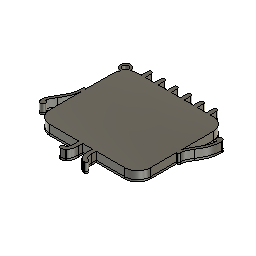
circuitree_waving (Autodesk Fusion 360 design; units mm, degrees)
Autodesk Fusion 360 part; units mm, degrees
sketch "Sketch5" plane through (0, 0, 0) normal (0, 0, 1) x (1, 0, 0)
  arc A0 (75.391183, -21.681566) -> (75.436997, -21.922178) centre (74.778364, -21.922919) cw
  arc A1 (74.022291, -23.163511) -> (75.391183, -21.681566) centre (74.021701, -21.789761) cw
  spline S0 degree 3 poles (74.022291, -23.163511) (74.037616, -23.163511) (74.052473, -23.161712) (74.067685, -23.161215) knots 0 0 0 0 1 1 1 1
  spline S1 degree 3 poles (74.067685, -23.161215) (73.783142, -26.92138) (72.233252, -29.438806) (70.849939, -31.685019) knots 0 0 0 0 1 1 1 1
  spline S2 degree 3 poles (70.849939, -31.685019) (69.634251, -33.659121) (68.485936, -35.52374) (68.528222, -37.805771) knots 0 0 0 0 1 1 1 1
  arc A2 (69.189293, -38.454952) -> (68.528222, -37.805771) centre (69.189495, -37.793567) cw
  spline S3 degree 3 poles (69.189293, -38.454952) (69.193491, -38.454952) (69.197625, -38.454888) (69.201824, -38.454827) knots 0 0 0 0 1 1 1 1
  arc A3 (69.85088, -37.781225) -> (69.201824, -38.454827) centre (69.189535, -37.793483) cw
  spline S4 degree 3 poles (69.85088, -37.781225) (69.815821, -35.887086) (70.817036, -34.261281) (71.976396, -32.378712) knots 0 0 0 0 1 1 1 1
  spline S5 degree 3 poles (71.976396, -32.378712) (73.518187, -29.875175) (75.436997, -26.759415) (75.436997, -21.922178) knots 0 0 0 0 1 1 1 1
  line L0 (24.056254, -13.559896) -> (62.230986, -13.559896)
  arc A4 (62.230986, -13.559896) -> (68.477474, -19.806384) centre (62.230986, -19.806384) cw
  line L1 (68.477474, -19.806384) -> (68.477474, -51.829553)
  arc A5 (68.477474, -51.829553) -> (62.230986, -58.076042) centre (62.230986, -51.829553) cw
  line L2 (62.230986, -58.076042) -> (24.056254, -58.076042)
  arc A6 (24.056254, -58.076042) -> (17.809766, -51.829553) centre (24.056254, -51.829553) cw
  line L3 (17.809766, -51.829553) -> (17.809766, -19.806384)
  arc A7 (17.809766, -19.806384) -> (24.056254, -13.559896) centre (24.056254, -19.806384) cw
  line L4 (24.056253, -13.890625) -> (62.230996, -13.890625)
  arc A8 (62.230996, -13.890625) -> (68.146753, -19.806383) centre (62.230994, -19.806384) cw
  line L5 (68.146753, -19.806383) -> (68.146753, -51.829528)
  arc A9 (68.146753, -51.829528) -> (62.23096, -57.745313) centre (62.230967, -51.829527) cw
  line L6 (62.23096, -57.745313) -> (24.05628, -57.745313)
  arc A10 (24.05628, -57.745313) -> (18.140495, -51.829528) centre (24.056281, -51.829527) cw
  line L7 (18.140495, -51.829528) -> (18.140495, -19.806383)
  arc A11 (18.140495, -19.806383) -> (24.056253, -13.890625) centre (24.056254, -19.806384) cw
  line L8 (62.23096, -13.229167) -> (60.771484, -13.229167)
  line L9 (60.771484, -13.229167) -> (60.771484, -9.921875)
  arc A12 (60.771484, -9.921875) -> (58.787109, -9.921875) centre (59.779297, -9.921875) cw
  line L10 (58.787109, -9.921875) -> (58.787109, -13.229167)
  line L11 (58.787109, -13.229167) -> (54.117215, -13.229167)
  line L12 (54.117215, -13.229167) -> (54.117215, -9.921875)
  arc A13 (54.117215, -9.921875) -> (52.13284, -9.921875) centre (53.125028, -9.921875) cw
  line L13 (52.13284, -9.921875) -> (52.13284, -13.229167)
  line L14 (52.13284, -13.229167) -> (47.462942, -13.229167)
  line L15 (47.462942, -13.229167) -> (47.462942, -9.921875)
  arc A14 (47.462942, -9.921875) -> (45.478567, -9.921875) centre (46.470754, -9.921875) cw
  line L16 (45.478567, -9.921875) -> (45.478567, -13.229167)
  line L17 (45.478567, -13.229167) -> (40.808673, -13.229167)
  line L18 (40.808673, -13.229167) -> (40.808673, -9.921875)
  arc A15 (40.808673, -9.921875) -> (38.824298, -9.921875) centre (39.816485, -9.921875) cw
  line L19 (38.824298, -9.921875) -> (38.824298, -13.229167)
  line L20 (38.824298, -13.229167) -> (34.154403, -13.229167)
  line L21 (34.154403, -13.229167) -> (34.154403, -9.921875)
  arc A16 (34.154403, -9.921875) -> (32.170028, -9.921875) centre (33.162216, -9.921875) cw
  line L22 (32.170028, -9.921875) -> (32.170028, -13.229167)
  line L23 (32.170028, -13.229167) -> (27.500132, -13.229167)
  line L24 (27.500132, -13.229167) -> (27.500132, -9.921875)
  arc A17 (27.500132, -9.921875) -> (25.515757, -9.921875) centre (26.507945, -9.921875) cw
  line L25 (25.515757, -9.921875) -> (25.515757, -13.229167)
  line L26 (25.515757, -13.229167) -> (24.056253, -13.229167)
  arc A18 (17.479036, -19.806383) -> (24.056253, -13.229167) centre (24.063698, -19.813828) cw
  line L27 (17.479036, -19.806383) -> (17.479036, -51.829528)
  arc A19 (24.056253, -58.406771) -> (17.479036, -51.829528) centre (24.063704, -51.822103) cw
  line L28 (24.056253, -58.406771) -> (38.764765, -58.406771)
  line L29 (38.764765, -58.406771) -> (38.764765, -60.788021)
  spline S6 degree 3 poles (38.764765, -60.788021) (38.764765, -63.974067) (37.304066, -64.152157) (37.137539, -64.161975) knots 0 0 0 0 1 1 1 1
  arc A20 (37.137539, -64.161975) -> (37.164035, -64.161458) centre (37.155354, -64.395884) cw
  line L30 (37.164035, -64.161458) -> (37.164035, -64.164296)
  spline S7 degree 3 poles (37.164035, -64.164296) (37.145314, -64.163243) (37.126787, -64.161458) (37.107813, -64.161458) knots 0 0 0 0 1 1 1 1
  arc A21 (37.107813, -64.161458) -> (37.107813, -66.145833) centre (37.107813, -65.153646) cw
  spline S8 degree 3 poles (37.107813, -66.145833) (37.126796, -66.145833) (37.145322, -66.144049) (37.164035, -66.142995) knots 0 0 0 0 1 1 1 1
  line L31 (37.164035, -66.142995) -> (37.164035, -66.145833)
  spline S9 degree 3 poles (37.164035, -66.145833) (37.267452, -66.145833) (38.200244, -66.124004) (39.099463, -65.367005) knots 0 0 0 0 1 1 1 1
  spline S10 degree 3 poles (39.099463, -65.367005) (40.194091, -64.445481) (40.74914, -62.904881) (40.74914, -60.788021) knots 0 0 0 0 1 1 1 1
  line L32 (40.74914, -60.788021) -> (40.74914, -58.406771)
  line L33 (40.74914, -58.406771) -> (45.703464, -58.406771)
  line L34 (45.703464, -58.406771) -> (45.703464, -60.788021)
  spline S11 degree 3 poles (45.703464, -60.788021) (45.703464, -62.909855) (46.272809, -64.453107) (47.395674, -65.374825) knots 0 0 0 0 1 1 1 1
  arc A22 (49.061952, -66.121372) -> (47.395674, -65.374825) centre (49.572732, -62.748496) cw
  arc A23 (49.278646, -66.145833) -> (49.061952, -66.121372) centre (49.281029, -65.152696) cw
  spline S12 degree 3 poles (49.278646, -66.145833) (49.286761, -66.145833) (49.294621, -66.144816) (49.302692, -66.144618) knots 0 0 0 0 1 1 1 1
  spline S13 degree 3 poles (49.302692, -66.144618) (49.327121, -66.145623) (49.344792, -66.145833) (49.354743, -66.145833) knots 0 0 0 0 1 1 1 1
  line L35 (49.354743, -66.145833) -> (49.354743, -66.14199)
  arc A24 (49.354743, -64.165302) -> (49.354743, -66.14199) centre (49.279616, -65.153646) cw
  line L36 (49.354743, -64.165302) -> (49.354743, -64.161458)
  spline S14 degree 2 poles (49.354743, -64.161458) (49.363205, -64.161067) (49.3791, -64.16185) knots 0 0 0 1 1 1
  spline S15 degree 3 poles (49.3791, -64.16185) (49.20598, -64.15254) (47.687839, -63.978782) (47.687839, -60.788021) knots 0 0 0 0 1 1 1 1
  line L37 (47.687839, -60.788021) -> (47.687839, -58.406771)
  line L38 (47.687839, -58.406771) -> (62.23096, -58.406771)
  arc A25 (68.808203, -51.829528) -> (62.23096, -58.406771) centre (62.223529, -51.822096) cw
  line L39 (68.808203, -51.829528) -> (68.808203, -19.806383)
  arc A26 (62.23096, -13.229167) -> (68.808203, -19.806383) centre (62.223535, -19.813835) cw
  arc A27 (68.146753, -51.829528) -> (62.23096, -57.745321) centre (62.224223, -51.82279) cw
  line L40 (62.23096, -57.745313) -> (24.056253, -57.745313)
  arc A28 (24.056253, -57.745313) -> (18.140495, -51.829528) centre (24.062991, -51.822817) cw
  line L41 (18.140495, -51.829528) -> (18.140495, -19.806383)
  arc A29 (18.140495, -19.806383) -> (24.056253, -13.890625) centre (24.062964, -19.813094) cw
  line L42 (24.056253, -13.890625) -> (62.23096, -13.890625)
  arc A30 (62.23096, -13.890625) -> (68.146745, -19.806384) centre (62.224249, -19.813121) cw
  line L43 (68.146753, -19.806383) -> (68.146753, -51.829528)
  line L44 (26.169527, -17.264063) -> (60.117719, -17.264063)
  arc A31 (60.117719, -17.264063) -> (64.058668, -21.205011) centre (60.117719, -21.205011) cw
  line L45 (64.058668, -21.205011) -> (64.058668, -50.166343)
  arc A32 (64.058668, -50.166343) -> (60.117719, -54.107292) centre (60.117719, -50.166343) cw
  line L46 (60.117719, -54.107292) -> (26.169527, -54.107292)
  arc A33 (26.169527, -54.107292) -> (22.228578, -50.166343) centre (26.169527, -50.166343) cw
  line L47 (22.228578, -50.166343) -> (22.228578, -21.205011)
  arc A34 (22.228578, -21.205011) -> (26.169527, -17.264063) centre (26.169527, -21.205011) cw
  arc A35 (35.849132, -30.780964) -> (34.745986, -27.830859) centre (35.848734, -29.099808) cw
  arc A36 (28.04587, -33.928121) -> (34.745986, -27.830859) centre (32.308182, -31.881942) cw
  line L48 (28.04587, -33.928121) -> (36.567568, -33.928121)
  arc A37 (36.819995, -30.471961) -> (36.567568, -33.928121) centre (32.289475, -31.878364) cw
  arc A38 (36.819995, -30.471961) -> (35.849132, -30.780964) centre (35.851181, -29.107714) cw
  arc A39 (58.026788, -30.051567) -> (55.75124, -27.637244) centre (56.688828, -29.033085) cw
  arc A40 (49.406254, -33.928105) -> (55.75124, -27.637244) centre (53.668615, -31.881919) cw
  line L49 (49.406254, -33.928105) -> (57.927956, -33.928105)
  arc A41 (58.026788, -30.051567) -> (57.927956, -33.928105) centre (53.655634, -31.879654) cw
  spline S16 degree 2 poles (43.30217, -39.892817) (43.240977, -39.892817) (43.179337, -39.891037) knots 0 0 0 1 1 1
  spline S17 degree 3 poles (43.179337, -39.891037) (42.500926, -39.871404) (41.52905, -39.714368) (40.751784, -39.077779) knots 0 0 0 0 1 1 1 1
  spline S18 degree 3 poles (40.751784, -39.077779) (39.974861, -38.441456) (39.575822, -37.488506) (39.56575, -36.245414) knots 0 0 0 0 1 1 1 1
  arc A42 (39.56575, -36.245414) -> (40.227208, -36.240048) centre (39.896479, -36.242731) cw
  spline S19 degree 3 poles (40.227208, -36.240048) (40.247652, -38.767191) (42.097568, -39.197979) (43.198478, -39.229841) knots 0 0 0 0 1 1 1 1
  spline S20 degree 3 poles (43.198478, -39.229841) (44.015228, -39.253414) (44.745343, -38.998132) (45.256168, -38.510953) knots 0 0 0 0 1 1 1 1
  spline S21 degree 3 poles (45.256168, -38.510953) (45.804649, -37.98789) (46.091966, -37.222692) (46.110251, -36.236641) knots 0 0 0 0 1 1 1 1
  arc A43 (46.110251, -36.236641) -> (46.440786, -35.912016) centre (46.440956, -36.242778) cw
  spline S22 degree 3 poles (46.440786, -35.912016) (46.442849, -35.912016) (46.44492, -35.912016) (46.447052, -35.91208) knots 0 0 0 0 1 1 1 1
  arc A44 (46.447052, -35.91208) -> (46.771584, -36.248849) centre (46.440911, -36.242753) cw
  spline S23 degree 3 poles (46.771584, -36.248849) (46.750263, -37.401585) (46.384075, -38.349331) (45.712669, -38.989602) knots 0 0 0 0 1 1 1 1
  spline S24 degree 3 poles (45.712669, -38.989602) (45.099448, -39.574426) (44.247235, -39.892817) (43.30217, -39.892817) knots 0 0 0 0 1 1 1 1
  arc A45 (17.585167, -34.040881) -> (16.26225, -34.040881) centre (16.923709, -34.040881) cw
  spline S25 degree 3 poles (16.26225, -34.040881) (16.26225, -38.503431) (14.528118, -41.319313) (12.998139, -43.803722) knots 0 0 0 0 1 1 1 1
  spline S26 degree 3 poles (12.998139, -43.803722) (11.782418, -45.777826) (10.634086, -47.642441) (10.676347, -49.924472) knots 0 0 0 0 1 1 1 1
  arc A46 (10.72089, -50.149402) -> (10.676347, -49.924472) centre (11.335073, -49.9109) cw
  arc A47 (12.119563, -48.672364) -> (10.72089, -50.149402) centre (12.090628, -50.045717) cw
  spline S27 degree 3 poles (12.119563, -48.672364) (12.416558, -47.271323) (13.22261, -45.962052) (14.124556, -44.497486) knots 0 0 0 0 1 1 1 1
  spline S28 degree 3 poles (14.124556, -44.497486) (15.666356, -41.993888) (17.585167, -38.878118) (17.585167, -34.040881) knots 0 0 0 0 1 1 1 1
  circle A48 centre (26.507945, -9.921875) radius 0.992187
  circle A49 centre (33.162216, -9.921875) radius 0.992188
  circle A50 centre (39.816485, -9.921875) radius 0.992188
  circle A51 centre (46.470754, -9.921875) radius 0.992188
  circle A52 centre (53.125028, -9.921875) radius 0.992188
  circle A53 centre (59.779297, -9.921875) radius 0.992188
  line L50 (49.279616, -65.153646) -> (37.107813, -65.153646)
  line L51 (49.279616, -65.153646) -> (50.270811, -65.153646)
  line L52 (37.107813, -65.153646) -> (36.116813, -65.153646)
  arc A54 (37.107813, -64.161458) -> (37.107812, -66.145833) centre (37.109001, -65.153646) ccw
  circle A55 centre (16.923709, -34.040881) radius 0.661458
  arc A56 (63.397668, -21.205011) -> (60.117719, -17.925062) centre (60.117719, -21.205011) ccw
  line L53 (63.397668, -21.205011) -> (63.397668, -50.166343)
  arc A57 (60.117719, -53.446292) -> (63.397668, -50.166343) centre (60.117719, -50.166343) ccw
  line L54 (60.117719, -53.446292) -> (26.169527, -53.446292)
  arc A58 (22.889578, -50.166343) -> (26.169527, -53.446292) centre (26.169527, -50.166343) ccw
  line L55 (22.889578, -50.166343) -> (22.889578, -21.205011)
  arc A59 (26.169527, -17.925063) -> (22.889578, -21.205011) centre (26.169527, -21.205011) ccw
  line L56 (26.169527, -17.925063) -> (60.117719, -17.925063)
  line L57 (19.407636, -15.157766) -> (14.171745, -9.921875)
  line L58 (19.407636, -15.157766) -> (26.812305, -15.157766) construction
  circle A60 centre (18.12249, -13.87262) radius 1.5
  circle A61 centre (18.12249, -13.87262) radius 2.632163
  dimension "d16" = 0.991
  dimension "d17" = 0.661
  dimension "d18" = 135
  dimension "d19" = 3
  dimension "d20" = 1.132163
  constraint concentric A17 A48
  constraint concentric A16 A49
  constraint concentric A15 A50
  constraint concentric A14 A51
  constraint concentric A13 A52
  constraint concentric A12 A53
  constraint parallel L50 L52
  constraint concentric A45 A55
  constraint horizontal L58
  measures "d18" angle of L57 L58
  measures "d19" diameter of A60
extrude "Extrude6" add sketch "Sketch5" along normal blind 1 contours A0 A1 S0 S1 S2 A2 S3 A3 S4 S5 L39 | S2 A2 L39 | S2 A2 L0 A4 L1 A5 L2 A6 L3 A7 L8 L9 A12 L10 L11 L12 A13 L13 L14 L15 A14 L16 L17 L18 A15 L19 L20 L21 A16 L22 L23 L24 A17 L25 L26 A18 L27 A19 L28 L29 S6 A20 L30 A21 S10 L32 L33 L34 S11 A24 L36 S14 S15 L37 L38 A25 L39 A26 S28 A48 A49 A50 A51 A52 A53 L50 L51 A55 A61 | A12 A53 | A13 A52 | S11 A22 A23 S12 S13 L35 A24 L50 L51 | A21 L31 S9 S10 L50 | A14 A51 | L30 S7 A21 L50 L52 A54 | A21 S8 L31 L50 L52 A54 | A15 A50 | L27 A45 S25 S26 A46 A47 S27 S28 A55 | L27 A45 S28 A55 | A16 A49 | L27 A45 A55 | L27 A45 A55 | A18 L57 A60 A61 | A7 A18 A61 | A17 A48 | A18 L57 A60 A61 | L0 A4 L1 A5 L2 A6 L3 A7 L4 A8 L5 A9 L6 A10 L7 A11 L40 L41 L42 L43 A61 | A7 A11 A61 | L44 A31 L45 A32 L46 A33 L47 A34 | A35 A36 L48 A37 A38 | A39 A40 L49 A41 | S16 S17 S18 A42 S19 S20 S21 A43 S22 A44 S23 S24 picked at (72.47717, -30.647685) picked at (68.629825, -37.746366) picked at (46.446039, -12.45654) picked at (59.536855, -10.146828) picked at (52.827051, -10.065373) picked at (48.984235, -65.765504) picked at (38.632064, -65.393434) picked at (46.78679, -10.019359) picked at (37.060784, -64.495605) picked at (37.060784, -65.811687) picked at (39.574044, -10.146828) picked at (14.736077, -42.550175) picked at (17.505546, -35.129378) picked at (32.864239, -10.065373) picked at (16.951293, -33.840096) picked at (17.494272, -34.132946) picked at (18.28669, -15.964023) picked at (19.569377, -15.319508) picked at (26.191909, -9.920774) picked at (20.215213, -14.059383) picked at (49.506067, -57.965799) picked at (19.784773, -15.416969) picked at (37.485591, -53.666625) picked at (33.184668, -32.790267) picked at (54.393033, -32.781223) picked at (46.523636, -36.606513) makes body 1 at (54.393033, -32.781223, 0) makes body 2 at (46.523636, -36.606513, 0) makes body 3 at (33.184668, -32.790267, 0) makes body 4 at (46.446039, -12.45654, 0) makes body 5 at (37.485591, -53.666625, 0)
extrude "Extrude7" add sketch "Sketch5" along normal blind 1 separate body contours A56 L53 A57 L54 A58 L55 A59 L56 picked at (43.196472, -48.928467) makes body 6
extrude "Extrude8" add sketch "Sketch5" along normal blind 1 separate body contours A11 A29 A61 | A11 A29 A61 | A11 A29 A61 | L4 L5 L6 L7 A27 L40 A28 L41 A29 L42 A30 L43 A61 | A29 A61 | A10 A28 | A8 A30 | A9 A27 picked at (18.829698, -17.062806) picked at (19.595584, -15.930483) picked at (21.312676, -14.579828) picked at (66.784058, -40.600751) picked at (19.913781, -15.663911) picked at (19.983937, -56.100755) picked at (66.5022, -15.734063) picked at (66.303306, -56.100756) makes body 7
extrude "Extrude9" add 28 faces at (72.47717, -30.647685, 1) (68.629825, -37.746366, 1) (46.446039, -12.45654, 1) (48.984235, -65.765504, 1) (38.632064, -65.393434, 1) (37.060784, -64.495605, 1) (17.505546, -35.129378, 1) (17.494272, -34.132946, 1) (19.569377, -15.319508, 1) (49.506067, -57.965799, 1) (26.191909, -9.920774, 1) (32.864239, -10.065373, 1) (39.574044, -10.146828, 1) (46.78679, -10.019359, 1) (52.827051, -10.065373, 1) (59.536855, -10.146828, 1) (37.060784, -65.811687, 1) (14.736077, -42.550175, 1) (16.951293, -33.840096, 1) (18.28669, -15.964023, 1) (20.215213, -14.059383, 1) (19.784773, -15.416969, 1) (66.784058, -40.600751, 1) (43.196472, -48.928467, 1) (33.184668, -32.790267, 1) (46.523636, -36.606513, 1) (54.393033, -32.781223, 1) (37.485591, -53.666625, 1) along direction (0, 0, 1) blind 4 separate body on bodies 1 2 3 4 5 6 7 makes body 8
scale "Scale1" factor 0.8 about (40.74914, -58.406771, 5) bodies 2 1 4 3 5 6 7 8
sketch "Sketch7" plane through (0, 0, 5) normal (0, 0, 1) x (-1, 0, 0)
  spline S0 degree 3 poles (-37.864086, 63.011692) (-37.854806, 63.011072) (-37.845511, 63.010521) (-37.836078, 63.010521) knots 0.37855773 0.37855773 0.37855773 0.37855773 1 1 1 1
  arc A0 (-37.836078, 63.010521) -> (-37.836078, 64.598021) centre (-37.837029, 63.804271) ccw
  spline S1 degree 3 poles (-37.836078, 64.598021) (-37.851264, 64.598021) (-37.866086, 64.596593) (-37.881056, 64.59575) knots 0 0 0 0 1 1 1 1
  spline S2 degree 3 poles (-37.881056, 64.598021) (-37.96379, 64.598021) (-38.710023, 64.580557) (-39.429398, 63.974958) knots 0 0 0 0 1 1 1 1
  spline S3 degree 3 poles (-39.429398, 63.974958) (-39.493804, 63.920737) (-39.555876, 63.863837) (-39.615607, 63.804271) knots 0 0 0 0 0.07354834 0.07354834 0.07354834 0.07354834
  ellipse E0 centre (-5.196266, 24.04137) end of major axis (-39.451013, 63.956585) minor radius 12.544277 (-39.615607, 63.804271) -> (-40.74914, 60.311771) ccw
  line L0 (-40.74914, 60.311771) -> (-40.74914, 58.406771)
  line L1 (-40.74914, 58.406771) -> (-44.712599, 58.406771)
  line L2 (-44.712599, 58.406771) -> (-44.712599, 60.311771)
  ellipse E1 centre (-81.171146, 23.902379) end of major axis (-45.987688, 63.914363) minor radius 12.727234 (-44.712599, 60.311771) -> (-45.869009, 63.804271) ccw
  spline S4 degree 3 poles (-45.869009, 63.804271) (-45.932228, 63.866121) (-45.998015, 63.925107) (-46.066367, 63.981214) knots 0.92390931 0.92390931 0.92390931 0.92390931 1 1 1 1
  arc A1 (-46.066367, 63.981214) -> (-47.39939, 64.578452) centre (-47.808014, 61.880151) ccw
  arc A2 (-47.39939, 64.578452) -> (-47.572745, 64.598021) centre (-47.574651, 63.803511) ccw
  spline S5 degree 3 poles (-47.572745, 64.598021) (-47.579236, 64.598021) (-47.585525, 64.597207) (-47.591981, 64.597049) knots 0 0 0 0 1 1 1 1
  spline S6 degree 3 poles (-47.591981, 64.597049) (-47.611525, 64.597853) (-47.625661, 64.598021) (-47.633623, 64.598021) knots 0 0 0 0 1 1 1 1
  arc A3 (-47.633623, 64.594946) -> (-47.652663, 63.015274) centre (-47.573521, 63.804271) ccw
  spline S7 degree 3 poles (-47.633872, 63.009393) (-47.428005, 62.990107) (-46.300099, 62.771683) (-46.300099, 60.311771) knots 0.03631457 0.03631457 0.03631457 0.03631457 1 1 1 1
  line L3 (-46.300099, 60.311771) -> (-46.300099, 58.406771)
  line L4 (-46.300099, 58.406771) -> (-57.934596, 58.406771)
  arc A4 (-57.934596, 58.406771) -> (-63.19639, 53.144976) centre (-57.928651, 53.139031) ccw
  line L5 (-63.19639, 53.144976) -> (-63.19639, 42.348539)
  arc A5 (-63.19639, 42.348539) -> (-63.501262, 42.445316) centre (-63.501424, 41.916208) ccw
  spline S8 degree 3 poles (-63.501262, 42.445316) (-63.504621, 42.445316) (-63.507928, 42.445264) (-63.511287, 42.445216) knots 0 0 0 0 1 1 1 1
  arc A6 (-63.511287, 42.445216) -> (-64.030532, 41.906334) centre (-63.501456, 41.916141) ccw
  spline S9 degree 3 poles (-64.030532, 41.906334) (-64.002485, 40.391023) (-64.803456, 39.090379) (-65.730945, 37.584324) knots 0 0 0 0 1 1 1 1
  spline S10 degree 3 poles (-65.730945, 37.584324) (-66.964378, 35.581494) (-68.499426, 33.088886) (-68.499426, 29.219097) knots 0 0 0 0 1 1 1 1
  arc A7 (-68.499426, 29.219097) -> (-68.462774, 29.026607) centre (-67.972519, 29.219689) ccw
  arc A8 (-68.462774, 29.026607) -> (-67.36766, 30.212163) centre (-67.367189, 29.113163) ccw
  spline S11 degree 3 poles (-67.36766, 30.212163) (-67.379921, 30.212163) (-67.391806, 30.210724) (-67.403976, 30.210327) knots 0 0 0 0 1 1 1 1
  spline S12 degree 3 poles (-67.403976, 30.210327) (-67.176341, 33.218458) (-65.93643, 35.232399) (-64.829779, 37.029369) knots 0 0 0 0 1 1 1 1
  spline S13 degree 3 poles (-64.829779, 37.029369) (-64.163928, 38.110615) (-63.523341, 39.150806) (-63.19639, 40.285215) knots 0 0 0 0 0.68464423 0.68464423 0.68464423 0.68464423
  line L6 (-63.19639, 40.285215) -> (-63.19639, 27.526461)
  arc A9 (-63.19639, 27.526461) -> (-57.934596, 22.264687) centre (-57.928656, 27.532422) ccw
  line L7 (-57.934596, 22.264688) -> (-56.767015, 22.264688)
  line L8 (-56.767015, 22.264688) -> (-56.767015, 19.618854)
  arc A10 (-56.767015, 19.618854) -> (-55.179515, 19.618854) centre (-55.973265, 19.618854) ccw
  line L9 (-55.179515, 19.618854) -> (-55.179515, 22.264688)
  line L10 (-55.179515, 22.264688) -> (-51.4436, 22.264688)
  line L11 (-51.4436, 22.264688) -> (-51.4436, 19.618854)
  arc A11 (-51.4436, 19.618854) -> (-49.8561, 19.618854) centre (-50.64985, 19.618854) ccw
  line L12 (-49.8561, 19.618854) -> (-49.8561, 22.264688)
  line L13 (-49.8561, 22.264688) -> (-46.120181, 22.264688)
  line L14 (-46.120181, 22.264688) -> (-46.120181, 19.618854)
  arc A12 (-46.120181, 19.618854) -> (-44.532681, 19.618854) centre (-45.326431, 19.618854) ccw
  line L15 (-44.532681, 19.618854) -> (-44.532681, 22.264688)
  line L16 (-44.532681, 22.264688) -> (-40.796766, 22.264688)
  line L17 (-40.796766, 22.264688) -> (-40.796766, 19.618854)
  arc A13 (-40.796766, 19.618854) -> (-39.209266, 19.618854) centre (-40.003016, 19.618854) ccw
  line L18 (-39.209266, 19.618854) -> (-39.209266, 22.264688)
  line L19 (-39.209266, 22.264688) -> (-35.473351, 22.264688)
  line L20 (-35.473351, 22.264688) -> (-35.473351, 19.618854)
  arc A14 (-35.473351, 19.618854) -> (-33.885851, 19.618854) centre (-34.679601, 19.618854) ccw
  line L21 (-33.885851, 19.618854) -> (-33.885851, 22.264688)
  line L22 (-33.885851, 22.264688) -> (-30.149934, 22.264688)
  line L23 (-30.149934, 22.264688) -> (-30.149934, 19.618854)
  arc A15 (-30.149934, 19.618854) -> (-28.562434, 19.618854) centre (-29.356184, 19.618854) ccw
  line L24 (-28.562434, 19.618854) -> (-28.562434, 22.264688)
  line L25 (-28.562434, 22.264688) -> (-27.394831, 22.264688)
  arc A16 (-27.394831, 22.264688) -> (-24.743595, 22.983973) centre (-27.400786, 27.532417) ccw
  arc A17 (-24.743595, 22.983973) -> (-22.852343, 24.875225) centre (-22.64782, 22.77945) ccw
  arc A18 (-22.852343, 24.875225) -> (-22.133057, 27.526461) centre (-27.400786, 27.532417) ccw
  line L26 (-22.133057, 27.526461) -> (-22.133057, 38.626573)
  arc A19 (-22.133057, 38.626573) -> (-21.159628, 38.914059) centre (-21.688795, 38.914059) ccw
  spline S14 degree 3 poles (-21.159628, 38.914059) (-21.159628, 42.484099) (-19.772323, 44.736804) (-18.548339, 46.724331) knots 0 0 0 0 1 1 1 1
  spline S15 degree 3 poles (-18.548339, 46.724331) (-17.575763, 48.303615) (-16.657097, 49.795307) (-16.690905, 51.620932) knots 0 0 0 0 1 1 1 1
  arc A20 (-16.690905, 51.620932) -> (-16.72654, 51.800876) centre (-17.217886, 51.610074) ccw
  arc A21 (-16.72654, 51.800876) -> (-17.845478, 50.619246) centre (-17.82233, 51.717927) ccw
  spline S16 degree 3 poles (-17.845478, 50.619246) (-18.083074, 49.498413) (-18.727916, 48.450996) (-19.449473, 47.279343) knots 0 0 0 0 1 1 1 1
  spline S17 degree 3 poles (-19.449473, 47.279343) (-20.510562, 45.55633) (-21.79486, 43.470881) (-22.133057, 40.458009) knots 0 0 0 0 0.86026828 0.86026828 0.86026828 0.86026828
  line L27 (-22.133057, 40.458009) -> (-22.133057, 53.144976)
  arc A22 (-22.133057, 53.144976) -> (-27.394831, 58.406771) centre (-27.400791, 53.139037) ccw
  line L28 (-27.394831, 58.406771) -> (-39.16164, 58.406771)
  line L29 (-39.16164, 58.406771) -> (-39.16164, 60.311771)
  spline S18 degree 3 poles (-39.16164, 60.311771) (-39.16164, 62.758164) (-38.085127, 62.98774) (-37.880797, 63.009187) knots 0 0 0 0 0.95980773 0.95980773 0.95980773 0.95980773
  circle A23 centre (-22.64782, 22.77945) radius 1.2
  line L30 (-16.72654, 51.800876) -> (-16.72654, 29.219689)
  line L31 (-16.72654, 29.219689) -> (-67.972519, 29.219689)
  constraint parallel L26 L30
  constraint perpendicular L30 L31
